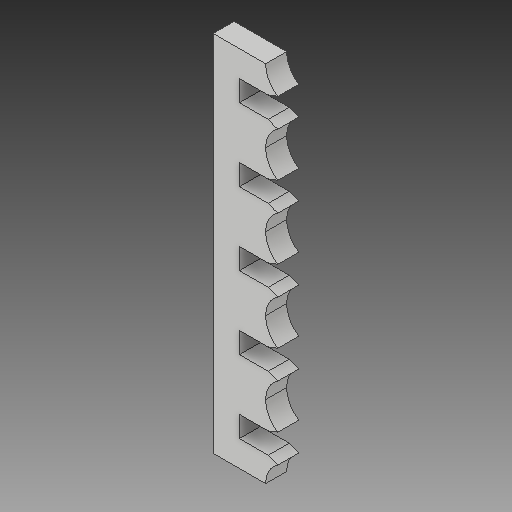
# Autodesk Inventor part: A
Saved by Autodesk Inventor 2019 (Build 230136000, 136)
## iProperties
Created: 2020-03-27
Part Number: A
Material: Generic
Document SubType Name: Modeling
Designer: Pulag
Density: 1 g/cm^3
Appearance: Default
Mass: 0.315499 g
Surface Area: 5.49611 cm^2
Volume: 0.315499 cm^3
Author: Pulag
Autodesk Inventor part; units mm, degrees
ref_plane "YZ Plane" through (0, 0, 0) normal (1, 0, 0) x (0, 1, 0)
ref_plane "XZ Plane" through (0, 0, 0) normal (0, 1, 0) x (-1, 0, 0)
ref_plane "XY Plane" through (0, 0, 0) normal (0, 0, 1) x (1, 0, 0)
sketch "Sketch1" plane through (0, 0, 0) normal (0, 0, 1) x (1, 0, 0)
  line L0 (0, 2.5) -> (-2.5, 2.5)
  arc A0 (1.1606, 4.6109) -> (0, 2.5) centre (2.5, 2.5) ccw
  line L1 (0, 2.5) -> (-1.5, 2.5)
  line L2 (-2.5, 4.9641) -> (0, 4.9641)
  line L3 (-5, 2.5) -> (-2.5, 2.5)
  line L4 (-5, 5.9641) -> (-5, 2.5)
  line L5 (-2.5, 5.9641) -> (-2.5, 4.9641)
  line L6 (0, 4.9641) -> (0.2479, 4.9641)
  arc A1 (0.2479, 4.9641) -> (1.1606, 4.6109) centre (2.5, 9.4282) ccw
  line L7 (0, 9.4282) -> (-2.5, 9.4282)
  arc A2 (0, 9.4282) -> (1.1606, 7.3173) centre (2.5, 9.4282) ccw
  line L8 (0, 9.4282) -> (-1.5, 9.4282)
  line L9 (-2.5, 6.9641) -> (0, 6.9641)
  line L10 (-5, 9.4282) -> (-2.5, 9.4282)
  line L11 (-5, 5.9641) -> (-5, 9.4282)
  line L12 (-2.5, 5.9641) -> (-2.5, 6.9641)
  line L13 (0, 6.9641) -> (0.2479, 6.9641)
  arc A3 (1.1606, 7.3173) -> (0.2479, 6.9641) centre (2.5, 2.5) ccw
  point P0 (0, 0)
  constraints: 28 end point, 8 point on circle, 4 centre point, 4 point on line, 1 horizontal, 1 parallel, 1 vertical
extrude "Extrusion1" add sketch "Sketch1" along normal blind 2
pattern_linear "Rectangular Pattern2" count 5 spacing 6.928 along (0, 1, 0) of "Extrusion1"
body "Solid1"
